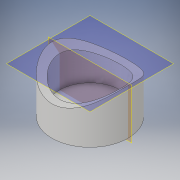
# Autodesk Inventor part: PistonTest1
Saved by Autodesk Inventor 2018 (Build 220112000, 112)
## iProperties
Created: 2019-08-30
Part Number: PistonTest1
Material: Generic
Document SubType Name: Modeling
Designer: 871357
Density: 1 g/cm^3
Appearance: Default
Author: 871357
Autodesk Inventor part; units mm, degrees
ref_plane "YZ Plane" through (0, 0, 0) normal (1, 0, 0) x (0, 1, 0)
ref_plane "XZ Plane" through (0, 0, 0) normal (0, 1, 0) x (-1, 0, 0)
sketch "Sketch1" plane through (0, 0, 0) normal (0, 1, 0) x (-1, 0, 0)
  circle A0 centre (0, 0) radius 6.35
  dimension "d0" = 12.7
  constraints: 1 centre point, 1 coincident
  measures "d0" diameter of A0
extrude "Extrusion1" add sketch "Sketch1" along normal blind 7.62
sketch "Sketch2" plane through (0, 0, 0) normal (0, 0, 1) x (1, 0, 0)
  line L0 (6.35, 7.62) -> (-6.35, 7.62) projected
  arc A0 (-6.35, 7.62) -> (6.35, 7.62) centre (0, 13.97) ccw
  line L1 (-6.35, 7.62) -> (-6.35, 5.08) construction
  line L2 (-6.35, 0) -> (-6.35, 7.62) construction
  point P0 (0, 0)
  dimension "d5" = 2.54
  dimension "d6" = 8.89
  constraints: 2 end point, 2 point on circle, 1 centre point, 1 point on line
  measures "d5" distance of L0.end L1.end
  measures "d6" vertical distance of L1.end A0.centre
extrude "Extrusion2" cut sketch "Sketch2" along normal mid plane 25.4
ref_plane "Work Plane1" through (0, 7.62, 0) normal (0, -1, 0) x (1, 0, 0)
sketch "Sketch3" plane through (0, 7.62, 0) normal (0, -1, 0) x (1, 0, 0)
  circle A0 centre (0, 0) radius 5.08
  dimension "d10" = 10.16
  constraints: 1 centre point, 1 coincident
  measures "d10" diameter of A0
extrude "Extrusion3" cut sketch "Sketch3" along normal blind 6.35
body "Solid1"
